Autodesk Fusion 360 part; units mm, degrees
(part 2 of 2)
extrude "Extrude1''''" add sketch "Sketch1 (4)" along normal blind 15 separate body contours L0 L1 L2 L3 L4 S0 S1 L5 L6 L7 L8 L9 L10 L11 L12 S2 S3 L13 S4 S5 L14 L15 L16 L17 L18 S6 L19 L20 L21 L22 L23 L24 L25 L26 S7 L27 L28 L29 L30 L31 L32 L33 L34 L35 L36 L37 S8 L38 L39 L40 L41 L42 L43 L44 L45 L46 L47 L48 L49 L50 L51 L52 L53 S9 L54 L55 L56 L57 L58 L59 L60 L61 L62 L63 S10 L64 L65 S11 L66 L67 S12 L68 L69 S13 L70 S14 L71 L72 L73 S15 L74 S16 L75 L76 L77 L78 L79 L80 L81 S17 L82 L83 S18 S19 L84 L85 S20 S21 S22 S23 L86 L87 L88 L89 S24 L90 L91 S25 L92 L93 S26 S27 S28 S29 L94 L95 S30 L96 S31 S32 S33 S34 S35 S36 S37 S38 L97 L98 S39 L99 S40 L100 S41 L101 S42 L102 S43 L103 S44 S45 S46 S47 S48 S49 S50 S51 S52 S53 S54 L104 L105 S55 L106 S56 L107 L108 L109 L110 L111 L112 L113 L114 L115 L116 L117 L118 L119 L120 L121 L122 L123 L124 L125 L126 L127 L128 L129 L130 L131 L132 L133 L134 L135 L136 L137 L138 L139 L140 L141 L142 L143 L144 L145 L146 L147 L148 L149 L150 L151 L152 L153 L154 L155 L156 L157 L158 L159 L160 L161 L162 L163 L164 L165 L166 L167 L168 L169 L170 L171 L172 L173 L174 L175 L176 L177 L178 L179 L180 L181 L182 L183 L184 L185 L186 L187 L188 L189 L190 S57 L191 L192 L193 L194 L195 L196 L197 S58 S59 L198 S60 S61 L199 L200 L201 L202 L203 L204 L205 L206 S62 S63 L207 L208 L209 L210 L211 S64 L212 L214 L216 | L187 L213 L215 L217 L218 L219 L220 L221 L222 L223 L224 L225 L226 L227 L228 L229 L230 L231 L232 L233 L234 L235 L236 makes body 5 in component "munich-background"
copy_body "Body->Comp2" [suppressed] in component "Component"
component "tampere-background" placed x (1, 0, 0) y (0, 1, 0) z (0, 0, 1) at (-57.5, -15.05, -36.875)
component "shelf" placed x (1, 0, 0) y (0, 1, 0) z (0, 0, 1) at (-57.5, -15.05, 23.125)
component "support-bar" placed x (1, 0, 0) y (0, 1, 0) z (0, 0, 1) at (-57.5, -60.8833, 25)
component "triangle-support" placed x (1, 0, 0) y (0, 1, 0) z (0, 0, 1) at (48.5, -0.05, 0)
component "triangle-support" placed x (1, 0, 0) y (0, 1, 0) z (0, 0, 1) at (280, 0, 0)
component "triangle-support" placed x (1, 0, 0) y (0, 1, 0) z (0, 0, 1) at (511.5, -0.05, 0)
component "munich-background" placed x (1, 0, 0) y (0, 1, 0) z (0, 0, 1) at (-57.5, -15.05, -36.8698)
component "tampere-background" placed x (1, 0, 0) y (0, 1, 0) z (0, 0, 1) at (-57.5, -15.05, 313.125)
component "shelf" placed x (1, 0, 0) y (0, 1, 0) z (0, 0, 1) at (-57.5, -15.05, 373.125)
component "support-bar" placed x (1, 0, 0) y (0, 1, 0) z (0, 0, 1) at (-57.5, -60.8833, 375)
component "triangle-support" placed x (1, 0, 0) y (0, 1, 0) z (0, 0, 1) at (48.5, -0.05, 350)
component "triangle-support" placed x (1, 0, 0) y (0, 1, 0) z (0, 0, 1) at (280, 0, 350)
component "triangle-support" placed x (1, 0, 0) y (0, 1, 0) z (0, 0, 1) at (511.5, -0.05, 350)
component "munich-background" placed x (1, 0, 0) y (0, 1, 0) z (0, 0, 1) at (-57.5, -15.05, 313.1302)
equation "thickness = 15 mm"
equation "width = 690 mm"
equation "depth = 160 mm"
equation "d12 = width"
equation "d13 = depth - thickness"
equation "d14 = width / 5"
equation "d16 = thickness"
equation "d17 = width / 5"
equation "d18 = thickness"
equation "d30 = width / 5"
equation "d31 = thickness"
equation "d32 = width / 5"
equation "d35 = thickness"
equation "d37 = thickness"
equation "d43 = thickness + snugness"
equation "d44 = depth * 0.98"
equation "d45 = load_diameter"
equation "d46 = load_diameter"
equation "d48 = depth / 3 + snugness"
equation "d50 = -thickness / 8"
equation "d52 = width"
equation "d53 = depth / 3"
equation "d54 = thickness"
equation "d60 = support_thickness"
equation "support_thickness = 10 mm"
equation "d63 = height"
equation "d64 = depth"
equation "d65 = support_thickness / 2"
equation "d66 = support_thickness / 2"
equation "d67 = depth / 4"
equation "d68 = height / 3.5 - snugness / 2"
equation "d71 = depth / 3 + snugness"
equation "d72 = thickness"
equation "d74 = thickness"
equation "height = 110 mm"
equation "d101 = width / 5"
equation "d102 = thickness"
equation "d104 = width / 5"
equation "d105 = thickness"
equation "d107 = thickness"
equation "load_diameter = 106 mm"
equation "d110 = height / 2 + thickness"
equation "d112 = thickness + snugness"
equation "d113 = width / 5"
equation "d115 = width / 5"
equation "d116 = thickness + snugness"
equation "d117 = width / 5"
equation "d118 = thickness + snugness"
equation "d119 = width / 5"
equation "d124 = thickness"
equation "d125 = ( height / 2 ) + thickness / 8 + snugness / 2"
equation "d126 = thickness"
equation "d127 = thickness + snugness"
equation "d128 = width / 5 / 2 - thickness / 2 - snugness / 2"
equation "d129 = height / 3.5 - snugness / 2 - thickness / 8"
equation "d130 = load_diameter"
equation "d131 = thickness + snugness"
equation "d132 = height / 3.5 - snugness / 2 - thickness / 8"
equation "d133 = load_diameter"
equation "d134 = height / 3.5 - snugness / 2 - thickness / 8"
equation "d135 = thickness + snugness"
equation "d136 = depth / 3 - thickness / 2 - snugness / 2"
equation "d145 = depth / 3 - thickness / 2 - snugness / 2"
equation "d158 = thickness + snugness"
equation "d159 = thickness + snugness"
equation "d160 = thickness + snugness"
equation "d165 = width / 5"
equation "d166 = width / 5"
equation "d167 = thickness"
equation "d168 = height / 2 + thickness"
equation "d169 = thickness"
equation "d170 = thickness * 2 - thickness / 8"
equation "d171 = load_diameter"
equation "d172 = thickness"
equation "d173 = thickness"
equation "d174 = thickness * 2 - thickness / 8"
equation "d175 = load_diameter"
equation "d176 = thickness"
equation "d177 = thickness * 2 - thickness / 8"
equation "d178 = thickness"
equation "d179 = width / 5 / 2 - thickness / 2"
equation "d180 = thickness"
equation "snugness = 0.1 mm"
equation "d186 = height / 5"
